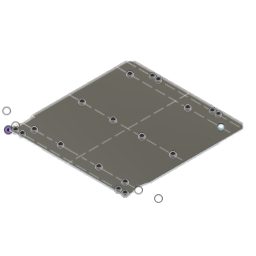
cr6-buildplate (Autodesk Fusion 360 design; units mm, degrees)
Autodesk Fusion 360 part; units mm, degrees
sketch "Sketch1" plane through (0, 0, 0) normal (0, 0, 1) x (1, 0, 0)
  line L0 (0, 0) -> (245, 0)
  line L1 (245, 255) -> (0, 255)
  line L2 (0, 27) -> (245, 27)
  line L3 (0, 227) -> (245, 227) construction
  line L4 (0, 127) -> (245, 127) construction
  circle A0 centre (27, 227) radius 4.5
  circle A1 centre (148, 227) radius 4.5
  circle A2 centre (217.5, 227) radius 4.5
  circle A3 centre (27, 127) radius 4.5
  circle A4 centre (92, 127) radius 4.5
  circle A5 centre (152, 127) radius 4.5
  circle A6 centre (217, 127) radius 4.5
  circle A7 centre (27, 27) radius 4.5
  circle A8 centre (82, 27) radius 4.5
  circle A9 centre (162, 27) radius 4.5
  circle A10 centre (217, 27) radius 4.5
  line L5 (0, 7) -> (245, 7) construction
  line L6 (0, 247) -> (245, 247) construction
  circle A11 centre (8, 7) radius 4
  circle A12 centre (22, 7) radius 4
  circle A13 centre (223, 7) radius 4
  circle A14 centre (237, 7) radius 4
  circle A15 centre (54, 247) radius 4
  circle A16 centre (66.5, 247) radius 4
  circle A17 centre (179.5, 247) radius 4
  circle A18 centre (192, 247) radius 4
  line L7 (122.5, 255) -> (122.5, 0) construction
  line L8 (0, 50) -> (4, 50) construction
  line L9 (4, 50) -> (4, 15) construction
  line L10 (4, 15) -> (0, 15) construction
  line L11 (0, 27) -> (0, 50) construction
  line L12 (4, 32.5) -> (0, 32.5) construction
  arc A19 (0, 15) -> (0, 50) centre (-36.2812, 32.5) ccw
  arc A20 (245, 50) -> (245, 15) centre (281.2812, 32.5) ccw
  line L13 (0, 255) -> (0, 50)
  line L14 (0, 32.5) -> (0, 27)
  line L15 (0, 15) -> (0, 0)
  line L16 (245, 0) -> (245, 15)
  line L17 (245, 50) -> (245, 255)
  line L18 (245, 50) -> (245, 15) construction
  line L19 (0, 50) -> (0, 15) construction
  dimension "d1" = 245
  dimension "d2" = 255
  dimension "d8" = 27
  dimension "d9" = 127
  dimension "d10" = 227
  dimension "d11" = 9
  dimension "d13" = 9
  dimension "d14" = 9
  dimension "d15" = 9
  dimension "d16" = 9
  dimension "d17" = 9
  dimension "d18" = 9
  dimension "d19" = 9
  dimension "d20" = 9
  dimension "d21" = 9
  dimension "d22" = 9
  dimension "d25" = 27
  dimension "d26" = 55
  dimension "d27" = 80
  dimension "d28" = 55
  dimension "d29" = 27
  dimension "d30" = 65
  dimension "d31" = 60
  dimension "d32" = 65
  dimension "d33" = 27
  dimension "d34" = 121
  dimension "d35" = 69.5
  dimension "d36" = 7
  dimension "d37" = 247
  dimension "d38" = 8
  dimension "d39" = 8
  dimension "d40" = 8
  dimension "d41" = 14
  dimension "d42" = 8
  dimension "d43" = 201
  dimension "d44" = 8
  dimension "d45" = 14
  dimension "d46" = 8
  dimension "d47" = 8
  dimension "d48" = 54
  dimension "d49" = 12.5
  dimension "d50" = 8
  dimension "d51" = 8
  dimension "d52" = 12.5
  dimension "d53" = 113
  dimension "d56" = 15
  dimension "d57" = 50
  dimension "d58" = 4
  constraint horizontal L0
  constraint vertical L16
  constraint horizontal L1
  constraint vertical L13
  constraint coincident L0.start L15.end
  constraint coincident L2.start L13
  constraint perpendicular L2 L16
  constraint coincident L3.start L13
  constraint coincident L3.end L16
  constraint perpendicular L3 L16
  constraint coincident L4.start L13
  constraint coincident L4.end L16
  constraint perpendicular L4 L16
  constraint coincident L3 A0.centre
  constraint coincident L3 A1.centre
  constraint coincident L4 A3.centre
  constraint coincident L4 A4.centre
  constraint coincident L4 A5.centre
  constraint coincident L4 A6.centre
  constraint coincident L2 A9.centre
  constraint coincident L2 A10.centre
  constraint coincident L2 A8.centre
  constraint coincident L2 A7.centre
  constraint coincident L5.start L13
  constraint coincident L5.end L16
  constraint perpendicular L5 L16
  constraint coincident L6.start L13
  constraint coincident L6.end L16
  constraint perpendicular L6 L16
  constraint coincident L5 A11.centre
  constraint coincident L5 A12.centre
  constraint coincident L5 A13.centre
  constraint coincident L5 A14.centre
  constraint coincident L6 A15.centre
  constraint coincident L6 A16.centre
  constraint coincident L6 A17.centre
  constraint coincident L6 A18.centre
  constraint midpoint L1 L7.start
  constraint midpoint L0 L7.end
  constraint coincident L10.end L13
  constraint horizontal L8
  constraint vertical L9
  constraint horizontal L10
  constraint vertical L11
  constraint coincident L8.start L11.end
  constraint midpoint L9 L12.start
  constraint coincident L12.start A19
  constraint tangent L9 A19
  constraint coincident L10.end A19.start
  constraint symmetric L7 L8.start A20.start
  constraint symmetric L7 L10.end A20.end
  constraint symmetric L7 A19 A20
  constraint collinear L13 L14
  constraint coincident L11 L12.end
  constraint collinear L14 L15
  constraint collinear L16 L17
  measures "d1" distance of L0.start L0.end
  measures "d2" distance of L0.start L1.end
  measures "d8" distance of L0 L2
  measures "d9" distance of L0 L4
  measures "d10" distance of L0 L3
  measures "d11" diameter of A0
  measures "d13" diameter of A1
  measures "d14" diameter of A2
  measures "d15" diameter of A3
  measures "d16" diameter of A4
  measures "d17" diameter of A5
  measures "d18" diameter of A6
  measures "d19" diameter of A7
  measures "d20" diameter of A8
  measures "d21" diameter of A9
  measures "d22" diameter of A10
  measures "d25" distance of L2.start A7.centre
  measures "d26" distance of A7.centre A8.centre
  measures "d27" distance of A8.centre A9.centre
  measures "d28" distance of A9.centre A10.centre
  measures "d29" distance of A3.centre L13
  measures "d30" distance of A3.centre A4.centre
  measures "d31" distance of A4.centre A5.centre
  measures "d32" distance of A5.centre A6.centre
  measures "d33" distance of A0.centre L13
  measures "d34" distance of A0.centre A1.centre
  measures "d35" distance of A1.centre A2.centre
  measures "d36" distance of L0 L5
  measures "d37" distance of L0 L6
  measures "d38" diameter of A11
  measures "d39" distance of A11.centre L13
  measures "d40" diameter of A12
  measures "d41" distance of A11.centre A12.centre
  measures "d42" diameter of A13
  measures "d43" distance of A12.centre A13.centre
  measures "d44" diameter of A14
  measures "d45" distance of A13.centre A14.centre
  measures "d46" diameter of A15
  measures "d47" diameter of A16
  measures "d48" distance of A15.centre L13
  measures "d49" distance of A15.centre A16.centre
  measures "d50" diameter of A17
  measures "d51" diameter of A18
  measures "d52" distance of A17.centre A18.centre
  measures "d53" distance of A16.centre A17.centre
  measures "d56" distance of L0 L10.end
  measures "d57" distance of L0 L8.start
  measures "d58" distance of L8.start L8.end
extrude "Extrude1" add sketch "Sketch1" along normal blind 2 contours L0 L2 A7 A8 A9 A10 A19 A20 L15 L16 | L1 L2 A7 A8 A9 A10 A19 A20 L13 L17
chamfer "Chamfer1" distance 10 angle 45 2 edges at (245, 255, 1) (0, 255, 1)
chamfer "Chamfer2" distance 2 angle 45 2 edges at (245, 0, 1) (0, 0, 1)
